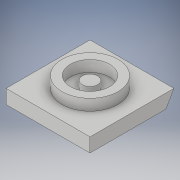
# Autodesk Inventor part: thumb_mount
Saved by Autodesk Inventor 2018 (Build 220112000, 112)
## iProperties
Created: 2017-11-07
Part Number: thumb_mount
Material: Generic
Document SubType Name: Modeling
Designer: rheal
Density: 1 g/cm^3
Appearance: Default
Author: rheal
Autodesk Inventor part; units mm, degrees
ref_plane "YZ Plane" through (0, 0, 0) normal (1, 0, 0) x (0, 1, 0)
ref_plane "XZ Plane" through (0, 0, 0) normal (0, 1, 0) x (-1, 0, 0)
ref_plane "XY Plane" through (0, 0, 0) normal (0, 0, 1) x (1, 0, 0)
sketch "Sketch1" plane through (0, 0, 0) normal (0, 1, 0) x (-1, 0, 0)
  line L0 (-15, 15) -> (15, 15)
  line L1 (15, 15) -> (15, -15)
  line L2 (15, -15) -> (-15, -15)
  line L3 (-15, -15) -> (-15, 15)
  line L4 (-15, 15) -> (15, -15) construction
  line L5 (15, 15) -> (-15, -15) construction
  point P0 (0, 0)
  dimension "d0" = 30
  dimension "d1" = 30
  constraints: 12 end point, 2 midpoint, 2 parallel, 1 horizontal, 1 perpendicular
  measures "d0" distance of L1.end L2.end
  measures "d1" distance of L0.end L1.end
extrude "Extrusion1" add sketch "Sketch1" along normal blind 5
sketch "Sketch2" plane through (0, 5, 0) normal (0, 1, 0) x (1, 0, 0)
  circle A0 centre (0, 0) radius 2.75
  dimension "d4" = 5.5
  constraints: 1 centre point, 1 coincident
  measures "d4" diameter of A0
extrude "Extrusion2" add sketch "Sketch2" along normal blind 2.5
sketch "Sketch3" plane through (0, 5, 0) normal (0, 1, 0) x (1, 0, 0)
  circle A0 centre (0, 0) radius 7
  circle A1 centre (0, 0) radius 10
  dimension "d7" = 14
  dimension "d8" = 20
  constraints: 2 centre point, 2 coincident
  measures "d7" diameter of A0
  measures "d8" diameter of A1
extrude "Extrusion3" add sketch "Sketch3" along normal blind 4
sketch "Sketch4" plane through (15, 0, 15) normal (1, 0, 0) x (0, 0, -1)
  line L0 (30, 5) -> (0, 5) projected
  line L1 (30, 0) -> (30, 5) projected
  line L2 (30, 5) -> (27.1132, 0)
  line L3 (30, 5) -> (39.3023, 5) construction
  line L4 (30, 0) -> (0, 0) projected
  line L5 (27.1132, 0) -> (30, 0)
  line L6 (30, 0) -> (30, 5)
  point P0 (15, 0)
  dimension "d12" = 120
  constraints: 8 end point, 1 collinear, 1 horizontal, 1 perpendicular, 1 point on line
  measures "d12" angle of L2 L3
extrude "Extrusion4" cut sketch "Sketch4" against normal blind 30
body "Solid1"
